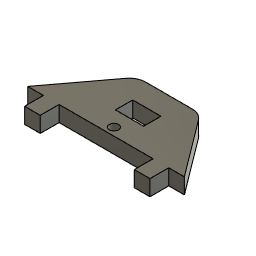
supporti_termice_1.0 (Autodesk Fusion 360 design; units mm, degrees)
Autodesk Fusion 360 part; units mm, degrees
sketch "Sketch1" plane through (0, 0, 0) normal (0, 1, 0) x (1, 0, 0)
  line L0 (0, 0) -> (-15, 0)
  line L1 (-15, 0) -> (-15, -6)
  line L2 (-15, -6) -> (-20, -6)
  line L3 (-20, -6) -> (-20, 0)
  line L4 (-20, 0) -> (-25, 0)
  line L5 (-7.5, 20) -> (0, 20)
  line L6 (0, 0) -> (15, 0)
  line L7 (15, 0) -> (15, -6)
  line L8 (15, -6) -> (20, -6)
  line L9 (20, -6) -> (20, 0)
  line L10 (20, 0) -> (25, 0)
  line L11 (7.5, 20) -> (0, 20)
  line L12 (-25, 0) -> (-11.5, 18)
  line L13 (25, 0) -> (11.5, 18)
  arc A0 (-7.5, 20) -> (-11.5, 18) centre (-7.5, 15) ccw
  arc A1 (11.5, 18) -> (7.5, 20) centre (7.5, 15) ccw
  line L14 (0, 13) -> (-4.5, 13)
  line L15 (-4.5, 13) -> (-4.5, 7.5)
  line L16 (-4.5, 7.5) -> (4.5, 7.5)
  line L17 (0, 13) -> (4.5, 13)
  line L18 (4.5, 13) -> (4.5, 7.5)
  circle A2 centre (0, 2.5) radius 1.5
  dimension "d1" = 5
  dimension "d6" = 2.5
  dimension "d7" = 3
  constraint coincident L0.start L6.start
  constraint horizontal L0
  constraint perpendicular L0 L1
  constraint perpendicular L1 L2
  constraint perpendicular L2 L3
  constraint perpendicular L3 L4
  constraint perpendicular L3 L5
  constraint tangent L12 A0
  constraint tangent L5 A0
  constraint tangent L13 A1
  constraint tangent L11 A1
  constraint equal A0 A1
  constraint horizontal L14
  constraint perpendicular L14 L15
  constraint perpendicular L15 L16
  constraint parallel L14 L17
  measures "d1" radius of A0
  measures "d6" distance of L0.start A2.centre
  measures "d7" diameter of A2
extrude "Extrude1" add sketch "Sketch1" along normal blind 5
